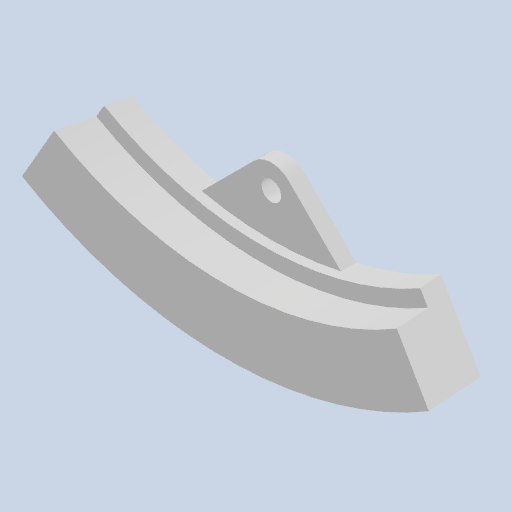
# Autodesk Inventor part: vzuh_karetka
Saved by Autodesk Inventor 2022 (Build 260153000, 153)
## iProperties
Created: 2024-09-10
Part Number: vzuh_karetka
Material: Типовые
Document SubType Name: Modeling
Designer: Andrey
Density: 1 g/cm^3
Appearance: По умолчанию
Author: Andrey
Autodesk Inventor part; units mm, degrees
ref_plane "YZ Plane" through (0, 0, 0) normal (1, 0, 0) x (0, 1, 0)
ref_plane "XZ Plane" through (0, 0, 0) normal (0, 1, 0) x (-1, 0, 0)
ref_plane "XY Plane" through (0, 0, 0) normal (0, 0, 1) x (1, 0, 0)
sketch "Эскиз1" plane through (0, 0, 0) normal (0, 0, 1) x (1, 0, 0)
  line L0 (-19.4221, 3.2482) -> (-17.0252, 13.9839) projected
  line L1 (17.0252, 13.9839) -> (19.4221, 3.2482) projected
  arc A0 (-41.5809, 15.0397) -> (41.5809, 15.0397) centre (0, 65) ccw projected
  line L2 (41.5809, 15.0397) -> (33.2647, 25.0318) projected
  arc A1 (-33.2647, 25.0318) -> (33.2647, 25.0318) centre (0, 65) ccw projected
  line L3 (-33.2647, 25.0318) -> (-41.5809, 15.0397) projected
  line L4 (-5.5, 11.5) -> (-5.5, 0.5) projected
  line L5 (5.5, 0.5) -> (5.5, 11.5) projected
  circle A2 centre (0, 65) radius 65
  circle A3 centre (0, 65) radius 52
  line L6 (-41.5809, 15.0397) -> (-33.2647, 25.0318)
  line L7 (20.5764, 3.3428) -> (0, 65)
  line L8 (-41.5809, 15.0397) -> (0, 65)
  line L9 (0, 65) -> (21.1137, 3.5247)
  line L10 (-32.5, 8.7083) -> (0, 65)
  line L11 (0, 65) -> (32.5, 8.7083)
  line L12 (0, 65) -> (0, 0)
  arc A4 (-39.7976, 13.9446) -> (-45.7382, 14.0977) centre (-42.8715, 10.0011) ccw projected
  line L13 (-45.7382, 14.0977) -> (-66.813, -0.6503) projected
  line L14 (-66.813, -0.6503) -> (-66.8135, -2.4814) projected
  line L15 (-66.8135, -2.4814) -> (-61.8135, -2.4828) projected
  line L16 (-61.8135, -2.4828) -> (-61.8127, 0.4976) projected
  arc A5 (-61.386, 1.3167) -> (-61.8127, 0.4976) centre (-60.8127, 0.4974) ccw projected
  line L17 (-61.386, 1.3167) -> (-46.2094, 11.9372) projected
  arc A6 (-40.3216, 11.8247) -> (-46.2094, 11.9372) centre (-43.3426, 7.8406) ccw projected
  arc A7 (-40.3216, 11.8247) -> (-21.0718, 1.6801) centre (0, 65) ccw projected
  line L18 (-21.0718, 1.6801) -> (-20.6332, 3.6423) projected
  arc A8 (-39.7976, 13.9446) -> (-20.6332, 3.6423) centre (0, 65) ccw projected
  circle A9 centre (0, 65) radius 64.7341
  arc A10 (-42.6225, 16.2781) -> (-20.6332, 3.6423) centre (0, 65) ccw projected
  line L19 (-42.6225, 16.2781) -> (0, 65)
  point P0 (0, 0)
  point P1 (0, 13)
  point P2 (-26, 19.9667)
  point P3 (-32.5, 8.7083)
  point P4 (32.5, 8.7083)
  point P5 (26, 19.9667)
  dimension "d23" = 0.5
  dimension "d25" = 60
  dimension "d26" = 30
  dimension "d42" = 60.135
  constraints: 16 end point, 8 point on circle, 3 coincident, 3 point on line, 2 centre point, 1 vertical, 1 vertical alignment, 2 other
  measures "d23" angle of L9 L7
  measures "d25" angle of L11 L10
  measures "d26" angle of L12 L10
  measures "d42" angle of L19 L9
extrude "Выдавливание1" add sketch "Эскиз1" along normal blind 10 contours L7 A9 L1 | L7 A1 L9 A9 | L1 A9 L12 A1 L7 | A9 L7 A0 L12 | A9 L9 A0 L7 | A9 L11 A0 L9 | L9 A1 L11 A9 | L12 A9 A8 L10 A1 | L12 A0 L18 A9 | A0 L10 A8 L18
sketch "Эскиз4" plane through (0, 0, 10) normal (0, 0, 1) x (1, 0, 0)
  arc A0 (-13.3607, 13.1952) -> (-9.9415, 12.4318) centre (0, 65) ccw projected
  circle A1 centre (0, 65) radius 53.5
  circle A2 centre (0, 65) radius 54.5
  line L0 (-26, 19.9667) -> (-32.5, 8.7083) projected
  arc A3 (-26, 19.9667) -> (-22.4589, 18.1001) centre (0, 65) ccw projected
  arc A4 (-26, 19.9667) -> (26, 19.9667) centre (0, 65) ccw projected
  arc A5 (22.4589, 18.1001) -> (26, 19.9667) centre (0, 65) ccw projected
  line L1 (32.5, 8.7083) -> (26, 19.9667) projected
  point P0 (0, 0)
  point P1 (-27.25, 17.8016)
  point P2 (27.25, 17.8016)
  dimension "d43" = 1
  constraints: 1 centre point, 1 coincident, 3 other
extrude "Выдавливание4" cut sketch "Эскиз4" against normal blind 5 contours A1 L0 A3 A4 L1 A0 | A0 A1 L1 A2 L0
draft "НаклГрань1" angle 10 pull direction (0, 0, -1) faces at (-30.75, 11.7394, 5) fixed edges at (-26.625, 18.8841, 5)
draft "НаклГрань2" angle 10 pull direction (0, 0, -1) faces at (30.75, 11.7394, 5) fixed edges at (26.625, 18.8841, 5)
sketch "Эскиз5" plane through (0, 0, 10) normal (0, 0, 1) x (1, 0, 0)
  arc A0 (-26, 19.9667) -> (26, 19.9667) centre (0, 65) ccw projected
  line L0 (-27.25, 17.8016) -> (-26, 19.9667) projected
  arc A1 (-27.25, 17.8016) -> (27.25, 17.8016) centre (0, 65) ccw projected
  line L1 (26, 19.9667) -> (27.25, 17.8016) projected
  point P0 (0, 0)
extrude "Выдавливание5" cut sketch "Эскиз5" against normal blind 6
sketch "Эскиз6" plane through (0, 0, 0) normal (0, 0, -1) x (-1, 0, 0)
  line L0 (-31.7335, 8.2727) -> (-25.2327, 19.5323) projected
  arc A0 (-25.2327, 19.5323) -> (25.2327, 19.5323) centre (0, 65) ccw projected
  arc A1 (-31.7335, 8.2727) -> (31.7335, 8.2727) centre (0, 65) ccw projected
  line L1 (25.2327, 19.5323) -> (31.7335, 8.2727) projected
  circle A2 centre (0, 20) radius 1.925 projected
  circle A3 centre (0, 20) radius 4 projected
  circle A4 centre (0, 20) radius 1.6
  circle A5 centre (0, 20) radius 4
  line L2 (-2.8284, 22.8284) -> (-11.3933, 14.2635)
  line L3 (2.8284, 22.8284) -> (11.3933, 14.2635)
  line L4 (0, 89.6007) -> (0, 9.3033) projected
  point P0 (0, 0)
  dimension "d50" = 3.2
  dimension "d51" = 8
  dimension "d52" = 45
  dimension "d53" = 45
  constraints: 4 end point, 4 point on circle, 2 centre point, 2 coincident, 2 tangent
  measures "d50" diameter of A4
  measures "d51" diameter of A5
  measures "d52" angle of L4 L2
  measures "d53" angle of L4 L3
extrude "Выдавливание6" add sketch "Эскиз6" against normal blind 2.5 contours L2 A3 L4 A0 | L4 A3 L3 A0 | A3 L4 A2 | L4 A2 A3 | L4 A4 A2 | A2 L4 A4
equation "\"d26\" = 0.5 * d25"
